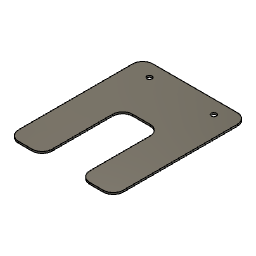
HammerHanger_steel v1 (Autodesk Fusion 360 design; units mm, degrees)
Autodesk Fusion 360 part; units mm, degrees
sketch "Sketch1" plane through (0, 0, 0) normal (0, 1, 0) x (1, 0, 0)
  line L0 (0, 0) -> (35.56, 0)
  line L1 (0, 0) -> (0, -76.2)
  line L2 (35.56, 0) -> (35.56, -76.2)
  line L3 (0, -76.2) -> (-31.75, -76.2)
  line L4 (35.56, -76.2) -> (67.31, -76.2)
  line L5 (-31.75, -76.2) -> (-31.75, 50.8)
  line L6 (67.31, -76.2) -> (67.31, 50.8)
  line L7 (-31.75, 50.8) -> (67.31, 50.8)
  line L8 (-31.75, 50.8) -> (-12.7, 50.8) construction
  line L9 (-12.7, 50.8) -> (-12.7, 38.1) construction
  line L10 (67.31, 50.8) -> (48.26, 50.8) construction
  line L11 (48.26, 50.8) -> (48.26, 38.1) construction
  circle A0 centre (48.26, 38.1) radius 2.3813
  circle A1 centre (-12.7, 38.1) radius 2.3813
  dimension "d2" = 76.2
  dimension "d3" = 76.2
  dimension "d4" = 31.75
  dimension "d5" = 31.75
  dimension "d6" = 127
  dimension "d7" = 127
  dimension "d8" = 19.05
  dimension "d9" = 4.7625
  dimension "d10" = 4.7625
  constraint coincident L0.start L1.start
  constraint horizontal L0
  constraint perpendicular L1 L3
  constraint perpendicular L2 L4
  constraint perpendicular L3 L5
  constraint perpendicular L4 L6
  constraint coincident L7 L8.end
  constraint perpendicular L6 L8
  constraint perpendicular L7 L9
  constraint perpendicular L6 L10
  constraint perpendicular L10 L11
  constraint coincident L11.end A0.centre
  constraint coincident L9.end A1.centre
  measures "d2" distance of L0.start L1.end
  measures "d3" distance of L0.end L2.end
  measures "d4" distance of L1.end L3.end
  measures "d5" distance of L2.end L4.end
  measures "d6" distance of L3.end L5.end
  measures "d7" distance of L4.end L6.end
  measures "d8" distance of L6.end L10.end
  measures "d9" diameter of A0
  measures "d10" diameter of A1
extrude "Extrude1" add sketch "Sketch1" along normal blind 1.5875 makes body 1
fillet "Fillet1" radius 9.525 8 edges at (0, 0.7937, 0) (35.56, 0.7937, 0) (-31.75, 0.7937, 76.2) (0, 0.7937, 76.2) (35.56, 0.7937, 76.2) (67.31, 0.7937, 76.2) (67.31, 0.7937, -50.8) (-31.75, 0.7937, -50.8) on bodies 1
copy_body "Body->Comp1" bodies 1 removing the originals makes body 2 in component "Component"
component "Component" placed x (1, 0, 0) y (0, 1, 0) z (0, 0, 1) at (0, 0, 0)
equation "d11 = ( 1 / 16 ) * 1 in"
